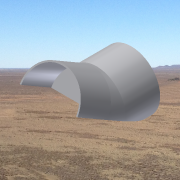
# Autodesk Inventor part: sup-angled
Saved by Autodesk Inventor 2013 SP2 (Build 170200200, 200)
## iProperties
Company: HERA Project
Created: 2013-06-12
Part Number: sup-angled
Material: PVC-Piping
Document SubType Name: Modeling
Designer: David DeBoer
Density: 1.4 g/cm^3
Description: Support angled connector
Mass: 54.0592 g
Surface Area: 239.655 cm^2
Volume: 38.6137 cm^3
Author: David DeBoer
Title: Support angled connector
Autodesk Inventor part; units mm, degrees
ref_plane "YZ Plane" through (0, 0, 0) normal (1, 0, 0) x (0, 1, 0)
sketch "Sketch1" plane through (0, 0, 0) normal (0, 0, 1) x (1, 0, 0)
  circle A0 centre (0, 0) radius 31.75
  dimension "d0" = 63.5
  constraints: 1 centre point, 1 coincident
  measures "d0" diameter of A0
extrude "Extrusion1" add sketch "Sketch1" along normal blind 38.1
sketch "Sketch2" plane through (0, 0, 38.1) normal (0, 0, 1) x (1, 0, 0)
  circle A0 centre (0, 0) radius 31.75 projected
  point P0 (0, 31.75)
  constraints: 1 vertical alignment, 1 other
ref_plane "Work Plane1" through (0, 31.75, 38.1) normal (0, 1, 0) x (-1, 0, 0)
sketch "Sketch3" plane through (0, 31.75, 38.1) normal (0, 1, 0) x (-1, 0, 0)
  line L0 (-11.7088, 2.54) -> (14.1872, 2.54) construction
  line L1 (31.75, 0) -> (-31.75, 0) projected
  point P0 (0, -38.1)
  dimension "d3" = 2.54
  constraints: 2 end point, 1 horizontal
  measures "d3" distance between parallel lines of L1 L0
ref_plane "Work Plane3" through (11.7088, 33.02, 42.8397) normal (0, 0.5, 0.8660254) x (-1, 0, 0)
ref_plane "Work Plane2" through (11.7088, 31.75, 40.64) normal (0, 0.5, 0.8660254) x (-1, 0, 0)
sketch "Sketch5" plane through (11.7088, 33.02, 42.8397) normal (0, 0.5, 0.8660254) x (-1, 0, 0)
  circle A0 centre (11.4573, 30.6064) radius 31.75
  line L0 (0.2164, -1.1436) -> (24.8554, -1.1436) construction
  point P0 (11.7088, 7.1763)
  dimension "d15" = 63.5
  dimension "d16" = 31.75
  constraints: 2 end point, 1 centre point, 1 horizontal
  measures "d15" diameter of A0
  measures "d16" distance from line of L0 A0.centre
extrude "Extrusion3" add sketch "Sketch5" along normal blind 38.1
loft "Loft1" add section 1 edges at (-31.75, 0, 38.1) section 2 edges at (32.0015, 6.5141, 58.1429)
sketch "Sketch6" plane through (0, 0, 0) normal (0, 0, -1) x (-1, 0, 0)
  circle A0 centre (0, 0) radius 31.75 projected
  circle A1 centre (0, 0) radius 30.1625
  dimension "d23" = 60.325
  constraints: 1 centre point, 1 coincident
  measures "d23" diameter of A1
extrude "Extrusion4" cut sketch "Sketch6" against normal blind 38.1 contours A1
sketch "Sketch7" plane through (0.2515, 25.5641, 91.1385) normal (0, 0.5, 0.8660254) x (1, 0, 0)
  circle A0 centre (0, 0) radius 31.75 projected
  circle A1 centre (0, 0) radius 30.1625
  point P0 (-0.2515, 23.4301)
  dimension "d26" = 60.325
  constraints: 1 centre point, 1 coincident
  measures "d26" diameter of A1
extrude "Extrusion5" cut sketch "Sketch7" against normal blind 38.1 contours A1
sketch "Sketch8" plane through (0.2515, 25.5641, 91.1385) normal (0, 0.5, 0.8660254) x (1, 0, 0)
  circle A0 centre (0, 0) radius 30.1625 projected
  circle A1 centre (0, 0) radius 31.75 projected
  point P0 (-0.2515, 23.4301)
  point P1 (0, -31.75)
  constraints: 1 vertical alignment, 1 other
ref_plane "Work Plane4" through (0.2515, -1.9323, 107.0135) normal (0, -0.8660254, 0.5) x (1, 0, 0)
sketch "Sketch9" plane through (0.2515, -1.9323, 107.0135) normal (0, -0.8660254, 0.5) x (1, 0, 0)
  line L0 (-48.3779, -109.4634) -> (50.7956, -109.4634)
  line L1 (50.7956, -109.4634) -> (50.7956, 8.7454)
  line L2 (50.7956, 8.7454) -> (-48.3779, 8.7454)
  line L3 (-48.3779, 8.7454) -> (-48.3779, -109.4634)
  point P0 (-0.2515, -91.7103)
  constraints: 8 end point, 2 parallel, 1 horizontal, 1 perpendicular
extrude "cut" cut sketch "Sketch9" against normal blind 31.75
body "Solid1"
